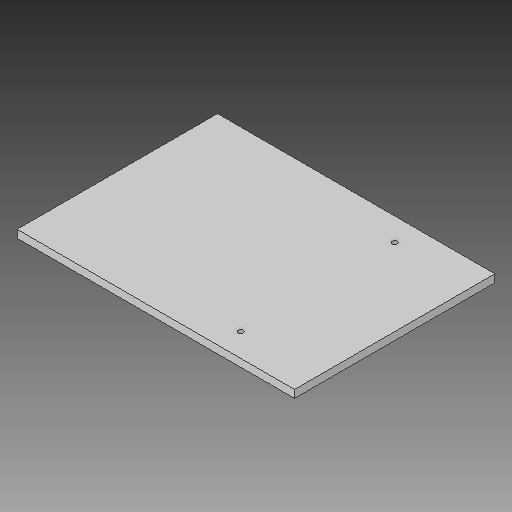
# Autodesk Inventor part: Plexiglass Hub Holding Plate
Saved by Autodesk Inventor 2019 (Build 230136000, 136)
## iProperties
Created: 2019-02-04
Part Number: Plexiglass Hub Holding Plate
Material: Generic
Document SubType Name: Modeling
Designer: mrhftc
Density: 1 g/cm^3
Appearance: Default
Author: mrhftc
Autodesk Inventor part; units mm, degrees
ref_plane "YZ Plane" through (0, 0, 0) normal (1, 0, 0) x (0, 1, 0)
ref_plane "XZ Plane" through (0, 0, 0) normal (0, 1, 0) x (-1, 0, 0)
ref_plane "XY Plane" through (0, 0, 0) normal (0, 0, 1) x (1, 0, 0)
sketch "Sketch1" plane through (0, 0, 0) normal (0, 1, 0) x (-1, 0, 0)
  line L0 (58.1245, 108.1229) -> (-170.4755, 108.1229)
  line L1 (-170.4755, 108.1229) -> (-170.4755, -56.9771)
  line L2 (-170.4755, -56.9771) -> (58.1245, -56.9771)
  line L3 (58.1245, -56.9771) -> (58.1245, 108.1229)
  line L4 (-106.9755, 33.9297) -> (-106.9755, 62.2792)
  circle A0 centre (-106.9755, 89.0729) radius 2.1
  circle A1 centre (-106.9755, -37.9271) radius 2.1
  point P0 (0, 0)
  dimension "d0" = 228.6
  dimension "d1" = 165.1
  dimension "d5" = 165.1
  dimension "d6" = 19.05
  dimension "d7" = 19.05
  dimension "d8" = 0
  dimension "d9" = 0
  dimension "d10" = 4.2
  dimension "d11" = 4.2
  constraints: 10 end point, 2 centre point, 2 parallel, 1 horizontal, 1 perpendicular, 1 vertical
  measures "d0" distance between parallel lines of L1 L3
  measures "d1" distance between parallel lines of L2 L0
  measures "d5" distance between parallel lines of L3 L4
  measures "d6" distance from line of L0 A0.centre
  measures "d7" distance from line of L2 A1.centre
  measures "d8" distance from line of L4 A1.centre
  measures "d9" distance from line of L4 A0.centre
  measures "d10" diameter of A1
  measures "d11" diameter of A0
extrude "Extrusion2" add sketch "Sketch1" along normal blind 6.35
body "Solid2"
